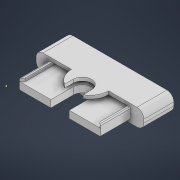
# Autodesk Inventor part: syringe_fitter
Saved by Autodesk Inventor 2022 (Build 260153000, 153)
## iProperties
Created: 2023-04-21
Part Number: syringe_fitter
Material: Generic
Document SubType Name: Modeling
Designer: Jakob Saugbjerg
Density: 1 g/cm^3
Appearance: Default
Author: Jakob Saugbjerg
Autodesk Inventor part; units mm, degrees
ref_plane "YZ Plane" through (0, 0, 0) normal (1, 0, 0) x (0, 1, 0)
ref_plane "XZ Plane" through (0, 0, 0) normal (0, 1, 0) x (-1, 0, 0)
ref_plane "XY Plane" through (0, 0, 0) normal (0, 0, 1) x (1, 0, 0)
sketch "Sketch13" plane through (0, 0, 0) normal (0, 0, 1) x (1, 0, 0)
  line L0 (0, 0) -> (63, 0)
  line L1 (63, 0) -> (63, 10)
  line L2 (63, 10) -> (0, 10)
  line L3 (0, 10) -> (0, 0)
  dimension "d38" = 63
  dimension "d39" = 10
  constraints: 8 end point, 2 parallel, 1 horizontal, 1 perpendicular
  measures "d38" distance of L2.end L1.end
  measures "d39" distance of L1.end L0.end
extrude "Extrusion8" add sketch "Sketch13" along normal blind 35
sketch "Sketch15" plane through (0, 10, 0) normal (0, 1, 0) x (1, 0, 0)
  line L0 (63, -35) -> (0, -35) projected
  line L1 (31.5, -35) -> (31.5, -22)
  circle A0 centre (31.5, -22) radius 5.4
  line L2 (44, -35) -> (26.1, -35)
  line L3 (26.1, -35) -> (26.1, -22)
  line L4 (36.9, -22) -> (36.9, -35)
  point P0 (0, 0)
  dimension "d42" = 13
  dimension "d43" = 10.8
  constraints: 8 end point, 2 point on circle, 2 point on line, 1 centre point, 1 coincident, 1 midpoint, 1 perpendicular, 1 vertical
  measures "d42" distance of L1.start L1.end
  measures "d43" diameter of A0
extrude "Extrusion9" cut sketch "Sketch15" against normal blind 35
sketch "Sketch16" plane through (0, 10, 0) normal (0, 1, 0) x (1, 0, 0)
  line L0 (0, -35) -> (26.1, -35) projected
  line L1 (0, -35) -> (63, -35)
  line L2 (63, -35) -> (63, -17.5)
  line L3 (63, -17.5) -> (0, -17.5)
  line L4 (0, -17.5) -> (0, -35)
  point P0 (0, 0)
  dimension "d46" = 63
  dimension "d47" = 17.5
  constraints: 8 end point, 2 parallel, 1 horizontal, 1 perpendicular
  measures "d46" distance of L3.end L2.end
  measures "d47" distance of L2.end L1.end
extrude "Extrusion10" cut sketch "Sketch16" against normal blind 2
sketch "Sketch17" plane through (0, 0, 0) normal (0, -1, 0) x (1, 0, 0)
  line L0 (0, 35) -> (26.1, 35) projected
  line L1 (0, 35) -> (63, 35)
  line L2 (63, 35) -> (63, 17.5)
  line L3 (63, 17.5) -> (0, 17.5)
  line L4 (0, 17.5) -> (0, 35)
  dimension "d71" = 63
  dimension "d72" = 17.5
  constraints: 8 end point, 2 parallel, 1 horizontal, 1 perpendicular
  measures "d71" distance of L2.end L3.end
  measures "d72" distance of L1.end L2.end
extrude "Extrusion11" cut sketch "Sketch17" against normal blind 2
sketch "Sketch19" plane through (0, 0, 35) normal (0, 0, 1) x (1, 0, 0)
  line L0 (26.1, 8) -> (0, 8) projected
  line L1 (9.5, 8) -> (53.5, 8)
  line L2 (53.5, 8) -> (53.5, 6.2)
  line L3 (53.5, 6.2) -> (9.5, 6.2)
  line L4 (9.5, 6.2) -> (9.5, 8)
  point P0 (0, 0)
  dimension "d68" = 1.8
  constraints: 8 end point, 2 parallel, 1 horizontal, 1 perpendicular, 1 point on line
  measures "d68" distance of L1.end L2.end
extrude "Extrusion12" cut sketch "Sketch19" against normal blind 33
fillet "Fillet5" radius 2 2 edges at (9.5, 7.1, 35) (53.5, 7.1, 35)
sketch "Sketch20" plane through (0, 0, 35) normal (0, 0, 1) x (1, 0, 0)
  line L0 (63, 8) -> (36.9, 8) projected
  line L1 (7.5, 2) -> (55.5, 2)
  line L2 (55.5, 2) -> (55.5, 8)
  line L3 (55.5, 8) -> (7.5, 8)
  line L4 (7.5, 8) -> (7.5, 2)
  line L5 (7.5, 2) -> (55.5, 8) construction
  line L6 (55.5, 2) -> (7.5, 8) construction
  line L7 (7.5, 8) -> (0, 8)
  line L8 (0, 8) -> (0, 2)
  line L9 (0, 2) -> (7.5, 2)
  line L10 (7.5, 2) -> (7.5, 8)
  line L11 (36.9, 2) -> (63, 2) projected
  line L12 (55.5, 8) -> (63, 8)
  line L13 (63, 8) -> (63, 2)
  line L14 (63, 2) -> (55.5, 2)
  line L15 (55.5, 2) -> (55.5, 8)
  point P0 (0, 0)
  point P1 (31.5, 5)
  point P2 (55.5, 2)
  dimension "d58" = 48
  constraints: 28 end point, 6 parallel, 3 horizontal, 3 perpendicular, 2 midpoint, 1 point on line
  measures "d58" distance of L3.end L2.end
extrude "Extrusion13" cut sketch "Sketch20" against normal blind 17.5 contours L13 L11 L2 L0 | L4 L9 L8 L7
fillet "Fillet6" radius 1 4 edges at (55.5, 2, 26.25) (55.5, 8, 26.25) (7.5, 8, 26.25) (7.5, 2, 26.25)
sketch "Sketch21" plane through (0, 0, 0) normal (0, 0, -1) x (-1, 0, 0)
  line L0 (-42.2521, 3.6325) -> (-44.1318, 3.6325)
  line L1 (-44.1318, 3.6325) -> (-44.1318, 4.0648)
  spline S0 degree 2 poles (-44.1318, 4.0648) (-43.9292, 4.255) (-43.5686, 4.6082) (-43.3957, 4.7984) knots 0 0 0 1 2 2 2
  spline S1 degree 2 poles (-43.3957, 4.7984) (-43.0474, 5.1812) (-42.793, 5.6407) (-42.793, 5.8852) knots 0 0 0 1 2 2 2
  spline S2 degree 2 poles (-42.793, 5.8852) (-42.793, 6.0136) (-42.8721, 6.2063) (-42.9437, 6.268) knots 0 0 0 1 2 2 2
  spline S3 degree 2 poles (-42.9437, 6.268) (-43.0153, 6.3298) (-43.2031, 6.3915) (-43.3167, 6.3915) knots 0 0 0 1 2 2 2
  spline S4 degree 2 poles (-43.3167, 6.3915) (-43.4254, 6.3915) (-43.6477, 6.3372) (-43.7489, 6.2952) knots 0 0 0 1 2 2 2
  spline S5 degree 2 poles (-43.7489, 6.2952) (-43.8354, 6.2606) (-43.9959, 6.1618) (-44.0453, 6.1272) knots 0 0 0 1 2 2 2
  line L2 (-44.0453, 6.1272) -> (-44.0676, 6.1272)
  line L3 (-44.0676, 6.1272) -> (-44.0676, 6.562)
  spline S6 degree 2 poles (-44.0676, 6.562) (-43.9416, 6.6237) (-43.4896, 6.7448) (-43.287, 6.7448) knots 0 0 0 1 2 2 2
  spline S7 degree 2 poles (-43.287, 6.7448) (-42.8597, 6.7448) (-42.3781, 6.2927) (-42.3781, 5.9074) knots 0 0 0 1 2 2 2
  spline S8 degree 2 poles (-42.3781, 5.9074) (-42.3781, 5.7271) (-42.4621, 5.4258) (-42.5362, 5.2973) knots 0 0 0 1 2 2 2
  spline S9 degree 2 poles (-42.5362, 5.2973) (-42.6103, 5.1639) (-42.8251, 4.9021) (-42.9437, 4.7762) knots 0 0 0 1 2 2 2
  spline S10 degree 2 poles (-42.9437, 4.7762) (-43.1364, 4.5662) (-43.6081, 4.1167) (-43.7489, 3.9857) knots 0 0 0 1 2 2 2
  line L4 (-43.7489, 3.9857) -> (-42.2521, 3.9857)
  line L5 (-42.2521, 3.9857) -> (-42.2521, 3.6325)
  line L6 (-37.8851, 3.6325) -> (-37.8851, 4.9565)
  spline S11 degree 2 poles (-37.8851, 4.9565) (-37.8851, 5.1145) (-37.9098, 5.3838) (-37.9493, 5.4579) knots 0 0 0 1 2 2 2
  spline S12 degree 2 poles (-37.9493, 5.4579) (-37.9889, 5.5394) (-38.1395, 5.6184) (-38.2704, 5.6184) knots 0 0 0 1 2 2 2
  spline S13 degree 2 poles (-38.2704, 5.6184) (-38.389, 5.6184) (-38.6607, 5.4727) (-38.804, 5.3344) knots 0 0 0 1 2 2 2
  spline S14 degree 2 poles (-38.804, 5.3344) (-38.8015, 5.2998) (-38.7966, 5.2035) (-38.7966, 5.1392) knots 0 0 0 1 2 2 2
  line L7 (-38.7966, 5.1392) -> (-38.7966, 3.6325)
  line L8 (-38.7966, 3.6325) -> (-39.1819, 3.6325)
  line L9 (-39.1819, 3.6325) -> (-39.1819, 4.9565)
  spline S15 degree 2 poles (-39.1819, 4.9565) (-39.1819, 5.1145) (-39.2066, 5.3838) (-39.2461, 5.4579) knots 0 0 0 1 2 2 2
  spline S16 degree 2 poles (-39.2461, 5.4579) (-39.2856, 5.5394) (-39.4363, 5.6184) (-39.5672, 5.6184) knots 0 0 0 1 2 2 2
  spline S17 degree 2 poles (-39.5672, 5.6184) (-39.6907, 5.6184) (-39.9649, 5.4628) (-40.0933, 5.3418) knots 0 0 0 1 2 2 2
  line L10 (-40.0933, 5.3418) -> (-40.0933, 3.6325)
  line L11 (-40.0933, 3.6325) -> (-40.4786, 3.6325)
  line L12 (-40.4786, 3.6325) -> (-40.4786, 5.9198)
  line L13 (-40.4786, 5.9198) -> (-40.0933, 5.9198)
  line L14 (-40.0933, 5.9198) -> (-40.0933, 5.6678)
  spline S18 degree 2 poles (-40.0933, 5.6678) (-39.9426, 5.8185) (-39.6462, 5.984) (-39.4684, 5.984) knots 0 0 0 1 2 2 2
  spline S19 degree 2 poles (-39.4684, 5.984) (-39.2659, 5.984) (-38.9522, 5.7987) (-38.8707, 5.5888) knots 0 0 0 1 2 2 2
  spline S20 degree 2 poles (-38.8707, 5.5888) (-38.6953, 5.7839) (-38.3643, 5.984) (-38.1716, 5.984) knots 0 0 0 1 2 2 2
  spline S21 degree 2 poles (-38.1716, 5.984) (-38.0234, 5.984) (-37.7814, 5.8926) (-37.6925, 5.7889) knots 0 0 0 1 2 2 2
  spline S22 degree 2 poles (-37.6925, 5.7889) (-37.6011, 5.6851) (-37.4998, 5.3739) (-37.4998, 5.1392) knots 0 0 0 1 2 2 2
  line L15 (-37.4998, 5.1392) -> (-37.4998, 3.6325)
  line L16 (-37.4998, 3.6325) -> (-37.8851, 3.6325)
  line L17 (-35.1632, 3.6325) -> (-36.9292, 3.6325)
  line L18 (-36.9292, 3.6325) -> (-36.9292, 6.6805)
  line L19 (-36.9292, 6.6805) -> (-36.5241, 6.6805)
  line L20 (-36.5241, 6.6805) -> (-36.5241, 3.9932)
  line L21 (-36.5241, 3.9932) -> (-35.1632, 3.9932)
  line L22 (-35.1632, 3.9932) -> (-35.1632, 3.6325)
  spline S23 degree 2 poles (-32.9476, 3.5782) (-33.1773, 3.5782) (-33.5749, 3.7017) (-33.7058, 3.7709) knots 0 0 0 1 2 2 2
  line L23 (-33.7058, 3.7709) -> (-33.7058, 4.2031)
  line L24 (-33.7058, 4.2031) -> (-33.6861, 4.2031)
  spline S24 degree 2 poles (-33.6861, 4.2031) (-33.6367, 4.1636) (-33.5033, 4.0697) (-33.3922, 4.0179) knots 0 0 0 1 2 2 2
  spline S25 degree 2 poles (-33.3922, 4.0179) (-33.2958, 3.9709) (-33.0587, 3.9018) (-32.9327, 3.9018) knots 0 0 0 1 2 2 2
  spline S26 degree 2 poles (-32.9327, 3.9018) (-32.8413, 3.9018) (-32.6314, 3.9438) (-32.582, 3.9783) knots 0 0 0 1 2 2 2
  spline S27 degree 2 poles (-32.582, 3.9783) (-32.5104, 4.0253) (-32.4461, 4.1315) (-32.4461, 4.2402) knots 0 0 0 1 2 2 2
  spline S28 degree 2 poles (-32.4461, 4.2402) (-32.4461, 4.376) (-32.5943, 4.5168) (-32.7845, 4.5637) knots 0 0 0 1 2 2 2
  spline S29 degree 2 poles (-32.7845, 4.5637) (-32.8586, 4.581) (-33.0958, 4.6304) (-33.197, 4.6576) knots 0 0 0 1 2 2 2
  spline S30 degree 2 poles (-33.197, 4.6576) (-33.4588, 4.7342) (-33.696, 5.0503) (-33.696, 5.2751) knots 0 0 0 1 2 2 2
  spline S31 degree 2 poles (-33.696, 5.2751) (-33.696, 5.5863) (-33.2291, 5.9741) (-32.8438, 5.9741) knots 0 0 0 1 2 2 2
  spline S32 degree 2 poles (-32.8438, 5.9741) (-32.6536, 5.9741) (-32.2683, 5.8802) (-32.1374, 5.8086) knots 0 0 0 1 2 2 2
  line L25 (-32.1374, 5.8086) -> (-32.1374, 5.3961)
  line L26 (-32.1374, 5.3961) -> (-32.1571, 5.3961)
  spline S33 degree 2 poles (-32.1571, 5.3961) (-32.3053, 5.5147) (-32.666, 5.6505) (-32.8512, 5.6505) knots 0 0 0 1 2 2 2
  spline S34 degree 2 poles (-32.8512, 5.6505) (-33.0414, 5.6505) (-33.3032, 5.49) (-33.3032, 5.3294) knots 0 0 0 1 2 2 2
  spline S35 degree 2 poles (-33.3032, 5.3294) (-33.3032, 5.1837) (-33.1476, 5.0429) (-32.9747, 4.9985) knots 0 0 0 1 2 2 2
  spline S36 degree 2 poles (-32.9747, 4.9985) (-32.8907, 4.9762) (-32.6783, 4.9318) (-32.5622, 4.9046) knots 0 0 0 1 2 2 2
  spline S37 degree 2 poles (-32.5622, 4.9046) (-32.3103, 4.8404) (-32.0534, 4.5464) (-32.0534, 4.292) knots 0 0 0 1 2 2 2
  spline S38 degree 2 poles (-32.0534, 4.292) (-32.0534, 4.1438) (-32.1695, 3.882) (-32.2831, 3.7857) knots 0 0 0 1 2 2 2
  spline S39 degree 2 poles (-32.2831, 3.7857) (-32.4041, 3.6844) (-32.7129, 3.5782) (-32.9476, 3.5782) knots 0 0 0 1 2 2 2
  line L27 (-29.8996, 5.9198) -> (-31.1296, 2.7903)
  line L28 (-31.1296, 2.7903) -> (-31.5421, 2.7903)
  line L29 (-31.5421, 2.7903) -> (-31.1321, 3.7437)
  line L30 (-31.1321, 3.7437) -> (-31.962, 5.9198)
  line L31 (-31.962, 5.9198) -> (-31.5471, 5.9198)
  line L32 (-31.5471, 5.9198) -> (-30.9221, 4.2253)
  line L33 (-30.9221, 4.2253) -> (-30.2997, 5.9198)
  line L34 (-30.2997, 5.9198) -> (-29.8996, 5.9198)
  line L35 (-28.3953, 5.5073) -> (-28.4151, 5.5073)
  spline S40 degree 2 poles (-28.4151, 5.5073) (-28.4595, 5.5196) (-28.5559, 5.5246) (-28.6226, 5.5246) knots 0 0 0 1 2 2 2
  spline S41 degree 2 poles (-28.6226, 5.5246) (-28.7782, 5.5246) (-29.0844, 5.3887) (-29.2228, 5.2553) knots 0 0 0 1 2 2 2
  line L36 (-29.2228, 5.2553) -> (-29.2228, 3.6325)
  line L37 (-29.2228, 3.6325) -> (-29.6081, 3.6325)
  line L38 (-29.6081, 3.6325) -> (-29.6081, 5.9198)
  line L39 (-29.6081, 5.9198) -> (-29.2228, 5.9198)
  line L40 (-29.2228, 5.9198) -> (-29.2228, 5.5789)
  spline S42 degree 2 poles (-29.2228, 5.5789) (-29.0128, 5.7666) (-28.6991, 5.9198) (-28.5509, 5.9198) knots 0 0 0 1 2 2 2
  spline S43 degree 2 poles (-28.5509, 5.9198) (-28.4916, 5.9198) (-28.4324, 5.9148) (-28.3953, 5.9074) knots 0 0 0 1 2 2 2
  line L41 (-28.3953, 5.9074) -> (-28.3953, 5.5073)
  line L42 (-27.7037, 3.6325) -> (-28.089, 3.6325)
  line L43 (-28.089, 3.6325) -> (-28.089, 5.9198)
  line L44 (-28.089, 5.9198) -> (-27.7037, 5.9198)
  line L45 (-27.7037, 5.9198) -> (-27.7037, 3.6325)
  line L46 (-27.6765, 6.3002) -> (-28.1137, 6.3002)
  line L47 (-28.1137, 6.3002) -> (-28.1137, 6.7003)
  line L48 (-28.1137, 6.7003) -> (-27.6765, 6.7003)
  line L49 (-27.6765, 6.7003) -> (-27.6765, 6.3002)
  line L50 (-25.3424, 3.6325) -> (-25.7277, 3.6325)
  line L51 (-25.7277, 3.6325) -> (-25.7277, 4.9367)
  spline S44 degree 2 poles (-25.7277, 4.9367) (-25.7277, 5.0948) (-25.7573, 5.3665) (-25.8018, 5.448) knots 0 0 0 1 2 2 2
  spline S45 degree 2 poles (-25.8018, 5.448) (-25.8487, 5.5344) (-26.0167, 5.6184) (-26.1599, 5.6184) knots 0 0 0 1 2 2 2
  spline S46 degree 2 poles (-26.1599, 5.6184) (-26.3032, 5.6184) (-26.607, 5.4653) (-26.7528, 5.3418) knots 0 0 0 1 2 2 2
  line L52 (-26.7528, 5.3418) -> (-26.7528, 3.6325)
  line L53 (-26.7528, 3.6325) -> (-27.1381, 3.6325)
  line L54 (-27.1381, 3.6325) -> (-27.1381, 5.9198)
  line L55 (-27.1381, 5.9198) -> (-26.7528, 5.9198)
  line L56 (-26.7528, 5.9198) -> (-26.7528, 5.6654)
  spline S47 degree 2 poles (-26.7528, 5.6654) (-26.5799, 5.821) (-26.2464, 5.984) (-26.0587, 5.984) knots 0 0 0 1 2 2 2
  spline S48 degree 2 poles (-26.0587, 5.984) (-25.7228, 5.984) (-25.3424, 5.5394) (-25.3424, 5.117) knots 0 0 0 1 2 2 2
  line L57 (-25.3424, 5.117) -> (-25.3424, 3.6325)
  spline S49 degree 2 poles (-24.7199, 3.267) (-24.6804, 3.2497) (-24.5297, 3.1953) (-24.4334, 3.1731) knots 0 0 0 1 2 2 2
  spline S50 degree 2 poles (-24.4334, 3.1731) (-24.3272, 3.1459) (-24.1469, 3.1138) (-24.0407, 3.1138) knots 0 0 0 1 2 2 2
  spline S51 degree 2 poles (-24.0407, 3.1138) (-23.8628, 3.1138) (-23.6158, 3.2077) (-23.5467, 3.2917) knots 0 0 0 1 2 2 2
  spline S52 degree 2 poles (-23.5467, 3.2917) (-23.48, 3.3757) (-23.4281, 3.5955) (-23.4281, 3.7363) knots 0 0 0 1 2 2 2
  line L58 (-23.4281, 3.7363) -> (-23.4281, 3.9363)
  spline S53 degree 2 poles (-23.4281, 3.9363) (-23.5837, 3.8005) (-23.8826, 3.6721) (-24.1074, 3.6721) knots 0 0 0 1 2 2 2
  spline S54 degree 2 poles (-24.1074, 3.6721) (-24.4976, 3.6721) (-24.9595, 4.2525) (-24.9595, 4.7984) knots 0 0 0 1 2 2 2
  spline S55 degree 2 poles (-24.9595, 4.7984) (-24.9595, 5.0824) (-24.799, 5.5221) (-24.6656, 5.6777) knots 0 0 0 1 2 2 2
  spline S56 degree 2 poles (-24.6656, 5.6777) (-24.5371, 5.8234) (-24.1839, 5.984) (-23.9962, 5.984) knots 0 0 0 1 2 2 2
  spline S57 degree 2 poles (-23.9962, 5.984) (-23.8184, 5.984) (-23.559, 5.9) (-23.4281, 5.8234) knots 0 0 0 1 2 2 2
  line L59 (-23.4281, 5.8234) -> (-23.4059, 5.9198)
  line L60 (-23.4059, 5.9198) -> (-23.0428, 5.9198)
  line L61 (-23.0428, 5.9198) -> (-23.0428, 3.8944)
  spline S58 degree 2 poles (-23.0428, 3.8944) (-23.0428, 3.3114) (-23.5491, 2.768) (-24.0703, 2.768) knots 0 0 0 1 2 2 2
  spline S59 degree 2 poles (-24.0703, 2.768) (-24.2383, 2.768) (-24.589, 2.8224) (-24.7397, 2.8668) knots 0 0 0 1 2 2 2
  line L62 (-24.7397, 2.8668) -> (-24.7397, 3.267)
  line L63 (-24.7397, 3.267) -> (-24.7199, 3.267)
  line L64 (-23.4281, 4.2525) -> (-23.4281, 5.5097)
  spline S60 degree 2 poles (-23.4281, 5.5097) (-23.5714, 5.5789) (-23.8134, 5.6382) (-23.9345, 5.6382) knots 0 0 0 1 2 2 2
  spline S61 degree 2 poles (-23.9345, 5.6382) (-24.2259, 5.6382) (-24.5618, 5.2084) (-24.5618, 4.8058) knots 0 0 0 1 2 2 2
  spline S62 degree 2 poles (-24.5618, 4.8058) (-24.5618, 4.4254) (-24.3074, 4.0277) (-24.0209, 4.0277) knots 0 0 0 1 2 2 2
  spline S63 degree 2 poles (-24.0209, 4.0277) (-23.8702, 4.0277) (-23.5541, 4.1463) (-23.4281, 4.2525) knots 0 0 0 1 2 2 2
  spline S64 degree 2 poles (-21.4916, 3.5807) (-22.04, 3.5807) (-22.6426, 4.1957) (-22.6426, 4.7638) knots 0 0 0 1 2 2 2
  spline S65 degree 2 poles (-22.6426, 4.7638) (-22.6426, 5.322) (-22.0573, 5.984) (-21.5855, 5.984) knots 0 0 0 1 2 2 2
  spline S66 degree 2 poles (-21.5855, 5.984) (-21.3731, 5.984) (-21.0445, 5.8605) (-20.9235, 5.7296) knots 0 0 0 1 2 2 2
  spline S67 degree 2 poles (-20.9235, 5.7296) (-20.8, 5.5987) (-20.6691, 5.2208) (-20.6691, 4.9466) knots 0 0 0 1 2 2 2
  line L65 (-20.6691, 4.9466) -> (-20.6691, 4.7366)
  line L66 (-20.6691, 4.7366) -> (-22.2524, 4.7366)
  spline S68 degree 2 poles (-22.2524, 4.7366) (-22.2524, 4.339) (-21.8522, 3.9166) (-21.4966, 3.9166) knots 0 0 0 1 2 2 2
  spline S69 degree 2 poles (-21.4966, 3.9166) (-21.3706, 3.9166) (-21.1261, 3.9734) (-21.0273, 4.0179) knots 0 0 0 1 2 2 2
  spline S70 degree 2 poles (-21.0273, 4.0179) (-20.9235, 4.0673) (-20.7803, 4.1537) (-20.7333, 4.1932) knots 0 0 0 1 2 2 2
  line L67 (-20.7333, 4.1932) -> (-20.7111, 4.1932)
  line L68 (-20.7111, 4.1932) -> (-20.7111, 3.7733)
  spline S71 degree 2 poles (-20.7111, 3.7733) (-20.7778, 3.7462) (-20.9803, 3.6671) (-21.0594, 3.6449) knots 0 0 0 1 2 2 2
  spline S72 degree 2 poles (-21.0594, 3.6449) (-21.1705, 3.6128) (-21.3533, 3.5807) (-21.4916, 3.5807) knots 0 0 0 1 2 2 2
  spline S73 degree 2 poles (-21.0445, 5.0306) (-21.0495, 5.1862) (-21.1137, 5.4134) (-21.1755, 5.49) knots 0 0 0 1 2 2 2
  spline S74 degree 2 poles (-21.1755, 5.49) (-21.2421, 5.5764) (-21.4521, 5.6678) (-21.6077, 5.6678) knots 0 0 0 1 2 2 2
  spline S75 degree 2 poles (-21.6077, 5.6678) (-21.7608, 5.6678) (-21.9757, 5.5764) (-22.0647, 5.4875) knots 0 0 0 1 2 2 2
  spline S76 degree 2 poles (-22.0647, 5.4875) (-22.1511, 5.3961) (-22.24, 5.1763) (-22.2524, 5.0306) knots 0 0 0 1 2 2 2
  line L69 (-22.2524, 5.0306) -> (-21.0445, 5.0306)
  point P0 (0, 0)
  point P1 (-44.3541, 6.7448)
  dimension "d38" = 63
  constraints: 1 other
emboss "Emboss3" sketch "Sketch21" operation cut depth 1 direction (0, 0, 1)
sketch "Sketch22" plane through (0, 0, 35) normal (0, 0, 1) x (1, 0, 0)
  point P0 (0, 0)
sketch "Sketch23" plane through (55.5, 3, 17.5) normal (1, 0, 0) x (0, 0, -1)
  line L0 (-15.5, 5) -> (0, 5) projected
  line L1 (-17.5, -1) -> (-17.5, 0) projected
  line L2 (0, 5) -> (-17.5, 5)
  line L3 (-17.5, 5) -> (-17.5, -1)
  line L4 (-17.5, -1) -> (0, -1)
  line L5 (0, -1) -> (0, 5)
  point P0 (17.5, -3)
  constraints: 8 end point, 2 parallel, 1 horizontal, 1 perpendicular
extrude "Extrusion14" cut sketch "Sketch23" against normal blind 0.2
sketch "Sketch24" plane through (7.5, 3, 17.5) normal (-1, 0, 0) x (0, 0, 1)
  line L0 (0, 5) -> (15.5, 5) projected
  line L1 (4.5, -1) -> (17.5, -1) projected
  line L2 (0, 5) -> (17.5, 5)
  line L3 (17.5, 5) -> (17.5, -1)
  line L4 (17.5, -1) -> (0, -1)
  line L5 (0, -1) -> (0, 5)
  point P0 (-17.5, -3)
  point P1 (3.5, -1)
  constraints: 8 end point, 2 parallel, 1 horizontal, 1 perpendicular
extrude "Extrusion15" cut sketch "Sketch24" against normal blind 0.2
fillet "Fillet7" radius 4 4 edges at (0, 10, 8.75) (0, 0, 8.75) (63, 10, 8.75) (63, 0, 8.75)
sketch "Sketch25" plane through (0, 0, 35) normal (0, 0, 1) x (1, 0, 0)
  point P0 (0, 0)
sketch "Sketch28" plane through (9.5, 6.2, 2) normal (0, 1, 0) x (1, 0, 0)
  circle A0 centre (22, -22) radius 5.7585
  line L0 (0, -15.5) -> (44, -15.5) projected
  circle A1 centre (22, -15.5) radius 10.85
  arc A2 (27.4, -20) -> (16.6, -20) centre (22, -20) ccw projected
  line L1 (27.4, -33) -> (27.4, -20) projected
  line L2 (16.6, -20) -> (27.4, -20)
  line L3 (27.4, -20) -> (27.4, -26.5)
  line L4 (27.4, -26.5) -> (16.6, -26.5)
  line L5 (16.6, -26.5) -> (16.6, -20)
  point P0 (-9.5, 2)
  point P1 (26.7504, -25.2548)
  point P2 (32.85, -15.5)
  point P3 (11.15, -15.5)
  point P4 (17.2496, -25.2548)
  point P5 (16.6, -24.9108)
  point P6 (27.4, -24.9108)
  point P7 (24.985, -15.5)
  point P8 (19.015, -15.5)
  dimension "d88" = 21.7
  constraints: 8 end point, 2 centre point, 2 midpoint, 2 parallel, 1 coincident, 1 horizontal, 1 perpendicular, 1 point on circle
  measures "d88" diameter of A1
extrude "Extrusion18" add sketch "Sketch28" along normal blind 3.8 contours A0 L1 | A0 A2 L0 A1 L1 | L5 A0 | A0 L5 A1 L0 A2
sketch "Sketch29" plane through (0, 0, 35) normal (0, 0, 1) x (1, 0, 0)
  line L0 (53.5, 6.2) -> (9.5, 6.2) projected
  line L1 (9.5, 8) -> (53.5, 8)
  line L2 (53.5, 8) -> (53.5, 6.2)
  line L3 (53.5, 6.2) -> (9.5, 6.2)
  line L4 (9.5, 6.2) -> (9.5, 8)
  point P0 (0, 0)
  constraints: 8 end point, 2 parallel, 1 horizontal, 1 perpendicular
extrude "Extrusion19" cut sketch "Sketch29" against normal blind 30
body "Solid2"
